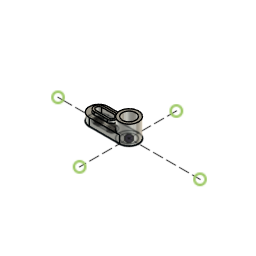
exercise03 (Autodesk Fusion 360 design; units mm, degrees)
Autodesk Fusion 360 part; units mm, degrees
sketch "草图1" plane through (0, 0, 0) normal (0, 0, 1) x (1, 0, 0)
  line L0 (-75, 0) -> (-70, 0) construction
  line L1 (-70, 0) -> (75, 0) construction
  line L2 (0, 50) -> (0, -52.1887) construction
  circle A0 centre (0, 0) radius 7
  circle A1 centre (0, 0) radius 10
  line L3 (-32, 5) -> (-18, 5)
  line L4 (-32, -5) -> (-18, -5)
  line L5 (-32, -3) -> (-18, -3)
  line L6 (-32, 3) -> (-18, 3)
  line L7 (-32, 10) -> (0, 10)
  line L8 (-32, -10) -> (0, -10)
  arc A2 (-32, 5) -> (-32, -5) centre (-32, 0) ccw
  arc A3 (-32, 3) -> (-32, -3) centre (-32, 0) ccw
  arc A4 (-18, -3) -> (-18, 3) centre (-18, 0) ccw
  arc A5 (-18, -5) -> (-18, 5) centre (-18, 0) ccw
  arc A6 (-32, 10) -> (-32, -10) centre (-32, 0) ccw
  dimension "d1" = 5
  dimension "d2" = 14
  dimension "d3" = 3
  dimension "d4" = 5
  dimension "d5" = 3
  dimension "d6" = 20
  dimension "d7" = 14
  dimension "d8" = 18
  dimension "d9" = 14
  constraint horizontal L0
  constraint parallel L0 L1
  constraint vertical L2
  constraint coincident L1 A0.centre
  constraint concentric A0 A1
  constraint horizontal L3
  constraint horizontal L4
  constraint parallel L3 L5
  constraint horizontal L6
  constraint tangent L4 A2
  constraint tangent L5 A3
  constraint concentric A2 A3
  constraint concentric A4 A5
  constraint collinear L0.start L1.end A4.centre
  constraint collinear A0.centre L0.start A2.centre
  constraint coincident A0.centre A1.centre
  constraint parallel L1 L7
  constraint parallel L1 L8
  constraint tangent L7 A6
  constraint tangent L8 A6
  constraint tangent A1 L8
  constraint equal L5 L6
  constraint equal L3 L4
  constraint coincident L2 L7.end
  constraint coincident L2 L8.end
  constraint concentric A2 A6
  constraint equal L3 L6
  measures "d1" radius of A2
  measures "d2" distance of A2.centre A4.centre
  measures "d3" radius of A3
  measures "d4" radius of A5
  measures "d5" radius of A4
  measures "d6" diameter of A1
  measures "d7" diameter of A0
  measures "d8" distance of A0.centre A4.centre
  measures "d9" distance of L3.start L3.end
extrude "拉伸1" add sketch "草图1" along normal blind 8 contours A1 L7 L8 A6
extrude "拉伸2" add sketch "草图1" along normal blind 20 contours A1
extrude "拉伸3" add sketch "草图1" along normal blind 11 contours L3 L4 A2 A5
